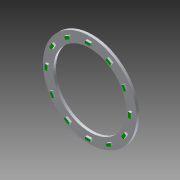
# Autodesk Inventor part: LED Ring
Saved by Autodesk Inventor 2014 SP1 (Build 180222100, 222)
## iProperties
Created: 2012-03-30
Part Number: LED Ring
Material: Generic
Document SubType Name: Modeling
Designer: Moses
Mass: 1.68561 g
Surface Area: 26.787 cm^2
Volume: 1.68561 cm^3
Density: 1 g/cm^3
Appearance: Smooth - White
Author: Moses
Autodesk Inventor part; units mm, degrees
ref_plane "YZ Plane" through (0, 0, 0) normal (1, 0, 0) x (0, 1, 0)
ref_plane "XZ Plane" through (0, 0, 0) normal (0, 1, 0) x (-1, 0, 0)
ref_plane "XY Plane" through (0, 0, 0) normal (0, 0, 1) x (1, 0, 0)
sketch "Sketch1" plane through (0, 0, 0) normal (0, 0, 1) x (1, 0, 0)
  circle A0 centre (0, 0) radius 22.225
  circle A1 centre (0, 0) radius 28.575
  line L0 (0, 0) -> (-22.225, 0) construction
  line L1 (-26.1937, 1.5875) -> (-24.6062, 1.5875)
  line L2 (-24.6062, 1.5875) -> (-24.6062, -1.5875)
  line L3 (-24.6062, -1.5875) -> (-26.1937, -1.5875)
  line L4 (-26.1937, -1.5875) -> (-26.1937, 1.5875)
  line L5 (-22.225, 0) -> (-28.575, 0) construction
  line L6 (-25.4, 1.5875) -> (-25.4, -1.5875) construction
  line L7 (-23.4782, -11.7221) -> (-22.1034, -10.9283)
  line L8 (-22.1034, -10.9283) -> (-20.5159, -13.6779)
  line L9 (-20.5159, -13.6779) -> (-21.8907, -14.4717)
  line L10 (-21.8907, -14.4717) -> (-23.4782, -11.7221)
  line L11 (-22.7908, -11.3252) -> (-21.2033, -14.0748) construction
  line L12 (-14.4717, -21.8907) -> (-13.6779, -20.5159)
  line L13 (-13.6779, -20.5159) -> (-10.9283, -22.1034)
  line L14 (-10.9283, -22.1034) -> (-11.7221, -23.4782)
  line L15 (-11.7221, -23.4782) -> (-14.4717, -21.8907)
  line L16 (-14.0748, -21.2033) -> (-11.3252, -22.7908) construction
  line L17 (-1.5875, -26.1938) -> (-1.5875, -24.6063)
  line L18 (-1.5875, -24.6063) -> (1.5875, -24.6063)
  line L19 (1.5875, -24.6063) -> (1.5875, -26.1938)
  line L20 (1.5875, -26.1938) -> (-1.5875, -26.1938)
  line L21 (-1.5875, -25.4) -> (1.5875, -25.4) construction
  line L22 (11.7221, -23.4782) -> (10.9283, -22.1034)
  line L23 (10.9283, -22.1034) -> (13.6779, -20.5159)
  line L24 (13.6779, -20.5159) -> (14.4717, -21.8907)
  line L25 (14.4717, -21.8907) -> (11.7221, -23.4782)
  line L26 (11.3252, -22.7908) -> (14.0748, -21.2033) construction
  line L27 (21.8907, -14.4717) -> (20.5159, -13.6779)
  line L28 (20.5159, -13.6779) -> (22.1034, -10.9283)
  line L29 (22.1034, -10.9283) -> (23.4782, -11.7221)
  line L30 (23.4782, -11.7221) -> (21.8907, -14.4717)
  line L31 (21.2033, -14.0748) -> (22.7908, -11.3252) construction
  line L32 (26.1938, -1.5875) -> (24.6063, -1.5875)
  line L33 (24.6063, -1.5875) -> (24.6063, 1.5875)
  line L34 (24.6063, 1.5875) -> (26.1938, 1.5875)
  line L35 (26.1938, 1.5875) -> (26.1938, -1.5875)
  line L36 (25.4, -1.5875) -> (25.4, 1.5875) construction
  line L37 (23.4782, 11.7221) -> (22.1034, 10.9283)
  line L38 (22.1034, 10.9283) -> (20.5159, 13.6779)
  line L39 (20.5159, 13.6779) -> (21.8907, 14.4717)
  line L40 (21.8907, 14.4717) -> (23.4782, 11.7221)
  line L41 (22.7908, 11.3252) -> (21.2033, 14.0748) construction
  line L42 (14.4717, 21.8907) -> (13.6779, 20.5159)
  line L43 (13.6779, 20.5159) -> (10.9283, 22.1034)
  line L44 (10.9283, 22.1034) -> (11.7221, 23.4782)
  line L45 (11.7221, 23.4782) -> (14.4717, 21.8907)
  line L46 (14.0748, 21.2033) -> (11.3252, 22.7908) construction
  line L47 (1.5875, 26.1937) -> (1.5875, 24.6063)
  line L48 (1.5875, 24.6063) -> (-1.5875, 24.6063)
  line L49 (-1.5875, 24.6063) -> (-1.5875, 26.1938)
  line L50 (-1.5875, 26.1938) -> (1.5875, 26.1937)
  line L51 (1.5875, 25.4) -> (-1.5875, 25.4) construction
  line L52 (-11.7221, 23.4782) -> (-10.9283, 22.1034)
  line L53 (-10.9283, 22.1034) -> (-13.6779, 20.5159)
  line L54 (-13.6779, 20.5159) -> (-14.4717, 21.8907)
  line L55 (-14.4717, 21.8907) -> (-11.7221, 23.4782)
  line L56 (-11.3252, 22.7908) -> (-14.0748, 21.2033) construction
  line L57 (-21.8907, 14.4717) -> (-20.5159, 13.6779)
  line L58 (-20.5159, 13.6779) -> (-22.1034, 10.9283)
  line L59 (-22.1034, 10.9283) -> (-23.4782, 11.7221)
  line L60 (-23.4782, 11.7221) -> (-21.8907, 14.4717)
  line L61 (-21.2033, 14.0748) -> (-22.7908, 11.3252) construction
  point P0 (-26.1937, 0)
  point P1 (-25.4, 0)
  point P2 (-22.6845, -13.0969)
  point P3 (-21.997, -12.7)
  point P4 (-13.0969, -22.6845)
  point P5 (-12.7, -21.997)
  point P6 (0, -26.1937)
  point P7 (0, -25.4)
  point P8 (13.0969, -22.6845)
  point P9 (12.7, -21.997)
  point P10 (22.6845, -13.0969)
  point P11 (21.997, -12.7)
  point P12 (26.1937, 0)
  point P13 (25.4, 0)
  point P14 (22.6845, 13.0969)
  point P15 (21.997, 12.7)
  point P16 (13.0969, 22.6845)
  point P17 (12.7, 21.997)
  point P18 (0, 26.1937)
  point P19 (0, 25.4)
  point P20 (-13.0969, 22.6845)
  point P21 (-12.7, 21.997)
  point P22 (-22.6845, 13.0969)
  point P23 (-21.997, 12.7)
  dimension "d0" = 44.45
  dimension "d1" = 57.15
  dimension "d2" = 3.175
  dimension "d3" = 1.5875
  dimension "d6" = 360
  constraints: 124 end point, 5 midpoint, 3 horizontal, 2 coincident, 2 horizontal alignment, 2 parallel, 2 point on line, 1 perpendicular, 161 other
  measures "d2" distance of L3.end L1.start
  measures "d3" distance of L1.start L1.end
extrude "Extrusion1" add sketch "Sketch1" against normal blind 1.5875 contours A1 | L1 L2 L3 L4 | L7 L8 L9 L10 | L12 L13 L14 L15 | L17 L18 L19 L20 | L22 L23 L24 L25 | L27 L28 L29 L30 | L32 L33 L34 L35 | L37 L38 L39 L40 | L42 L43 L44 L45 | L47 L48 L49 L50 | L52 L53 L54 L55 | L57 L58 L59 L60
extrude "Extrusion2" add sketch "Sketch1" along normal blind 1.27 contours L1 L2 L3 L4 | L7 L8 L9 L10 | L12 L13 L14 L15 | L17 L18 L19 L20 | L22 L23 L24 L25 | L27 L28 L29 L30 | L32 L33 L34 L35 | L37 L38 L39 L40 | L42 L43 L44 L45 | L47 L48 L49 L50 | L52 L53 L54 L55 | L57 L58 L59 L60
body "Solid1"
